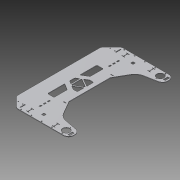
# Autodesk Inventor part: Shell
Saved by Autodesk Inventor 2015 (Build 190159000, 159)
## iProperties
Created: 2011-09-21
Part Number: Shell
Document SubType Name: Modeling
Designer: user
Density: 0.899 g/cm^3
Material: Polypropylene
Appearance: Smooth - White
Author: user
Autodesk Inventor part; units mm, degrees
ref_plane "YZ Plane" through (0, 0, 0) normal (1, 0, 0) x (0, 1, 0)
ref_plane "XZ Plane" through (0, 0, 0) normal (0, 1, 0) x (-1, 0, 0)
ref_plane "XY Plane" through (0, 0, 0) normal (0, 0, 1) x (1, 0, 0)
sketch "Profile" plane through (0, 0, 0) normal (0, 1, 0) x (-1, 0, 0)
  line L0 (-100, 0) -> (-164.5111, -37.2455)
  line L1 (-200.5386, -133.0137) -> (-188.6082, -71.0879)
  line L2 (-225.0872, -153.2843) -> (-230, -153.2843)
  arc A0 (-164.5111, -37.2455) -> (-188.6082, -71.0879) centre (-139.5111, -80.5468) ccw
  arc A1 (-225.0872, -153.2843) -> (-200.5386, -133.0137) centre (-225.0872, -128.2843) ccw
  arc A2 (-255, -128.2843) -> (-230, -153.2843) centre (-230, -128.2843) ccw
  line L3 (-100, 0) -> (0, 0)
  line L4 (-153, 47) -> (-143, 47)
  line L5 (-143, 47) -> (-143, 53)
  line L6 (-143, 53) -> (-153, 53)
  line L7 (-153, 53) -> (-153, 47)
  line L8 (-249.1421, 105.8579) -> (-210.8579, 144.1421)
  line L9 (-196.7157, 150) -> (0, 150)
  arc A3 (-249.1421, 105.8579) -> (-255, 91.7157) centre (-235, 91.7157) ccw
  arc A4 (-196.7157, 150) -> (-210.8579, 144.1421) centre (-196.7157, 130) ccw
  line L10 (0, 0) -> (0, 150) construction
  line L11 (-255, -128.2843) -> (-255, 91.7157)
  line L12 (-224.5, 102.5) -> (-221.5, 102.5)
  line L13 (-221.5, 102.5) -> (-221.5, 99.5)
  line L14 (-221.5, 99.5) -> (-224.5, 99.5)
  line L15 (-224.5, 99.5) -> (-224.5, 102.5)
  line L16 (-224.5, 124.5) -> (-221.5, 124.5)
  line L17 (-221.5, 124.5) -> (-221.5, 121.5)
  line L18 (-221.5, 121.5) -> (-224.5, 121.5)
  line L19 (-224.5, 121.5) -> (-224.5, 124.5)
  line L20 (-40, 25) -> (-40, 38.7438)
  arc A5 (-39.2646, 41.354) -> (-40, 38.7438) centre (-35, 38.7438) ccw
  arc A6 (-40, 25) -> (-35, 20) centre (-35, 25) ccw
  line L21 (-5.7735, 20) -> (-35, 20)
  line L22 (-114, 0) -> (-115, 0)
  line L23 (-116, 1) -> (-116, 11)
  line L24 (-115, 12) -> (-114, 12)
  line L25 (-113, 11) -> (-113, 1)
  line L26 (-211, 12) -> (-221, 12)
  line L27 (-222, 11) -> (-222, 1)
  line L28 (-221, 0) -> (-211, 0)
  line L29 (-210, 1) -> (-210, 11)
  arc A7 (-113, 11) -> (-114, 12) centre (-114, 11) ccw
  arc A8 (-114, 0) -> (-113, 1) centre (-114, 1) ccw
  arc A9 (-116, 1) -> (-115, 0) centre (-115, 1) ccw
  arc A10 (-115, 12) -> (-116, 11) centre (-115, 11) ccw
  arc A11 (-221, 12) -> (-222, 11) centre (-221, 11) ccw
  arc A12 (-210, 11) -> (-211, 12) centre (-211, 11) ccw
  arc A13 (-211, 0) -> (-210, 1) centre (-211, 1) ccw
  arc A14 (-222, 1) -> (-221, 0) centre (-221, 1) ccw
  line L30 (-247.5, -142.5) -> (-215.5, -142.5) construction
  line L31 (100, 0) -> (164.5111, -37.2455)
  line L32 (200.5386, -133.0137) -> (188.6082, -71.0879)
  line L33 (225.0872, -153.2843) -> (230, -153.2843)
  arc A15 (188.6082, -71.0879) -> (164.5111, -37.2455) centre (139.5111, -80.5468) ccw
  arc A16 (200.5386, -133.0137) -> (225.0872, -153.2843) centre (225.0872, -128.2843) ccw
  arc A17 (230, -153.2843) -> (255, -128.2843) centre (230, -128.2843) ccw
  line L34 (100, 0) -> (0, 0)
  line L35 (153, 47) -> (143, 47)
  line L36 (143, 47) -> (143, 53)
  line L37 (143, 53) -> (153, 53)
  line L38 (153, 53) -> (153, 47)
  line L39 (249.1421, 105.8579) -> (210.8579, 144.1421)
  arc A18 (255, 91.7157) -> (249.1421, 105.8579) centre (235, 91.7157) ccw
  arc A19 (210.8579, 144.1421) -> (196.7157, 150) centre (196.7157, 130) ccw
  line L40 (255, -128.2843) -> (255, 91.7157)
  line L41 (224.5, 102.5) -> (221.5, 102.5)
  line L42 (221.5, 102.5) -> (221.5, 99.5)
  line L43 (221.5, 99.5) -> (224.5, 99.5)
  line L44 (224.5, 99.5) -> (224.5, 102.5)
  line L45 (224.5, 124.5) -> (221.5, 124.5)
  line L46 (221.5, 124.5) -> (221.5, 121.5)
  line L47 (221.5, 121.5) -> (224.5, 121.5)
  line L48 (224.5, 121.5) -> (224.5, 124.5)
  line L49 (40, 25) -> (40, 38.7438)
  arc A20 (40, 38.7438) -> (39.2646, 41.354) centre (35, 38.7438) ccw
  arc A21 (35, 20) -> (40, 25) centre (35, 25) ccw
  line L50 (5.7735, 20) -> (35, 20)
  line L51 (114, 0) -> (115, 0)
  line L52 (116, 1) -> (116, 11)
  line L53 (115, 12) -> (114, 12)
  line L54 (113, 11) -> (113, 1)
  line L55 (211, 12) -> (221, 12)
  line L56 (222, 11) -> (222, 1)
  line L57 (221, 0) -> (211, 0)
  line L58 (210, 1) -> (210, 11)
  arc A22 (114, 12) -> (113, 11) centre (114, 11) ccw
  arc A23 (113, 1) -> (114, 0) centre (114, 1) ccw
  arc A24 (115, 0) -> (116, 1) centre (115, 1) ccw
  arc A25 (116, 11) -> (115, 12) centre (115, 11) ccw
  arc A26 (222, 11) -> (221, 12) centre (221, 11) ccw
  arc A27 (211, 12) -> (210, 11) centre (211, 11) ccw
  arc A28 (210, 1) -> (211, 0) centre (211, 1) ccw
  arc A29 (221, 0) -> (222, 1) centre (221, 1) ccw
  line L59 (-247.5, -142.5) -> (-247.5, 96.5) construction
  line L60 (-215.5, -142.5) -> (-215.5, 96.5) construction
  line L61 (-215.5, 96.5) -> (-247.5, 96.5) construction
  circle A30 centre (-250, -117.5) radius 2.5
  circle A31 centre (-250, -67.5) radius 2.5
  circle A32 centre (-250, -17.5) radius 2.5
  circle A33 centre (-250, 32.5) radius 2.5
  circle A34 centre (-250, 82.5) radius 2.5
  circle A35 centre (250, -117.5) radius 2.5
  circle A36 centre (250, -67.5) radius 2.5
  circle A37 centre (250, -17.5) radius 2.5
  circle A38 centre (250, 32.5) radius 2.5
  circle A39 centre (250, 82.5) radius 2.5
  line L62 (-173, 47) -> (-163, 47)
  line L63 (-163, 47) -> (-163, 53)
  line L64 (-163, 53) -> (-173, 53)
  line L65 (-173, 53) -> (-173, 47)
  line L66 (-193, 47) -> (-183, 47)
  line L67 (-183, 47) -> (-183, 53)
  line L68 (-183, 53) -> (-193, 53)
  line L69 (-193, 53) -> (-193, 47)
  line L70 (173, 47) -> (163, 47)
  line L71 (163, 53) -> (173, 53)
  line L72 (173, 53) -> (173, 47)
  line L73 (163, 47) -> (163, 53)
  line L74 (193, 47) -> (183, 47)
  line L75 (183, 53) -> (193, 53)
  line L76 (193, 53) -> (193, 47)
  line L77 (183, 47) -> (183, 53)
  line L78 (196.7157, 150) -> (0, 150)
  line L79 (-25.4034, 64) -> (25.4034, 64)
  line L80 (-25.4034, 64) -> (0, 20)
  line L81 (25.4034, 64) -> (0, 20)
  line L82 (-28.3745, 59.146) -> (-5.7735, 20)
  line L83 (28.3745, 59.146) -> (5.7735, 20)
  line L84 (-39.2646, 41.354) -> (-28.3745, 59.146)
  line L85 (39.2646, 41.354) -> (28.3745, 59.146)
  line L86 (-22.343, 69) -> (22.343, 69)
  line L87 (22.343, 69) -> (14.9249, 81.1195)
  line L88 (8, 85) -> (-8, 85)
  line L89 (-14.9249, 81.1195) -> (-22.343, 69)
  arc A40 (-8, 85) -> (-14.9249, 81.1195) centre (-8, 76.8809) ccw
  arc A41 (14.9249, 81.1195) -> (8, 85) centre (8, 76.8809) ccw
  point P0 (-184.2881, -48.6637)
  point P1 (-204.4439, -153.2843)
  point P2 (-205, 150)
  point P3 (-223, 121.5)
  point P4 (-223, 102.5)
  point P5 (0, 20)
  point P6 (-116, 12)
  point P7 (-116, 0)
  point P8 (-113, 12)
  point P9 (-210, 12)
  point P10 (-222, 12)
  point P11 (-210, 0)
  point P12 (184.2881, -48.6637)
  point P13 (204.4439, -153.2843)
  point P14 (205, 150)
  point P15 (223, 121.5)
  point P16 (223, 102.5)
  point P17 (40, 20)
  point P18 (40, 40)
  point P19 (116, 12)
  point P20 (116, 0)
  point P21 (113, 12)
  point P22 (210, 12)
  point P23 (222, 12)
  point P24 (210, 0)
  point P25 (-114.5, 0)
  point P26 (0, 85)
  dimension "d595" = 12
  dimension "d646" = 100
  dimension "d649" = 5
  dimension "d653" = 50
  dimension "d658" = 239
  dimension "d659" = 32
  dimension "d660" = 5
  dimension "d665" = 150
  dimension "d666" = 50
  dimension "d668" = 220
  dimension "d673" = 13
  dimension "d675" = 3
  dimension "d677" = 1
  dimension "d678" = 12
  dimension "d679" = 43
  dimension "d680" = 6
  dimension "d681" = 10
  dimension "d682" = 47
  dimension "d686" = 20
  dimension "d691" = 25
  dimension "d695" = 20
  dimension "d699" = 3
  dimension "d703" = 3
  dimension "d708" = 5
  dimension "d710" = 150
  dimension "d711" = 58.2843
  dimension "d713" = 5
  dimension "d714" = 33
  dimension "d716" = 45
  dimension "d717" = 130.905
  dimension "d720" = 54.4614
  dimension "d722" = 155
  dimension "d738" = 25
  dimension "d759" = 20
  dimension "d760" = 80
  dimension "d762" = 60
  dimension "d767" = 5
  dimension "d768" = 5
  dimension "d769" = 148.53
  dimension "d774" = 5
  dimension "d775" = 16
  dimension "d777" = 65
  dimension "d779" = 16
  dimension "d780" = 21.354
  dimension "d796" = 25
  dimension "d798" = 3
  dimension "d799" = 25.5
  dimension "d800" = 30.5
  constraints: 180 end point, 83 symmetric about line, 64 point on circle, 42 centre point, 39 point on line, 35 tangent, 13 parallel, 12 horizontal, 10 equal radius, 8 perpendicular, 6 collinear, 6 horizontal alignment, 4 midpoint, 4 vertical, 2 coincident, 45 other
  measures "d595" distance of point (-116, 0) point (-116, 12)
  measures "d646" distance of L0.start L3.end
  measures "d649" diameter of A30
  measures "d653" distance of A30.centre A31.centre
  measures "d658" distance of L30.end L60.end
  measures "d659" distance of L30.start L30.end
  measures "d660" radius of A6
  measures "d665" angle of L3 L0
  measures "d666" radius of A0
  measures "d668" distance of L11.start L11.end
  measures "d673" distance from line of L0.start L25
  measures "d675" distance between parallel lines of L25 L23
  measures "d677" radius of A7
  measures "d678" distance between parallel lines of L29 L27
  measures "d679" distance from line of L0.start L5
  measures "d680" distance of L4.end L5.end
  measures "d681" distance of L5.end L6.end
  measures "d682" distance between parallel lines of L3 L4
  measures "d686" distance of L4.end L62.end
  measures "d691" radius of A2
  measures "d695" radius of A4
  measures "d699" distance of L16.end L17.end
  measures "d703" distance between parallel lines of L61 L14
  measures "d708" radius of A5
  measures "d710" distance between parallel lines of L3 L9
  measures "d711" distance from line of L9 L11.end
  measures "d713" distance from line of L11 A30.centre
  measures "d714" distance between parallel lines of L11 L27
  measures "d716" angle of L8 L9
  measures "d717" angle of L1 L0
  measures "d720" horizontal distance of L11.start L1.start
  measures "d722" distance from line of L0.start L11
  measures "d738" distance from line of L30 A30.centre
  measures "d759" distance between parallel lines of L3 L21
  measures "d760" distance between parallel lines of L49 L20
  measures "d762" angle of L81 L79
  measures "d767" distance between parallel lines of L82 L80
  measures "d768" distance between parallel lines of L81 L83
  measures "d769" angle of L20 L84
  measures "d774" distance between parallel lines of L79 L86
  measures "d775" distance between parallel lines of L86 L88
  measures "d777" distance between parallel lines of L50 L88
  measures "d779" distance of L88.start L88.end
  measures "d780" distance from line of L21 L84.start
  measures "d796" distance between parallel lines of L14 L16
  measures "d798" distance of L16.start L16.end
  measures "d799" distance between parallel lines of L9 L16
  measures "d800" distance between parallel lines of L11 L19
extrude "Extrusion22" add sketch "Profile" along normal blind 3
sketch "Sketch40" plane through (0, 3, 0) normal (0, 1, 0) x (1, 0, 0)
  line L0 (255, -91.7157) -> (255, 128.2843) projected
  line L1 (-255, 128.2843) -> (-255, -91.7157) projected
  circle A0 centre (207.5, 114.5) radius 1.5
  circle A1 centre (250, 117.5) radius 2.5 projected
  circle A2 centre (-250, 117.5) radius 2.5 projected
  line L2 (0, 0) -> (0, 165.3372) construction
  circle A3 centre (228, 114.5) radius 17.5
  circle A4 centre (-207.5, 114.5) radius 1.5
  circle A5 centre (-228, 114.5) radius 17.5
  dimension "d742" = 5
  dimension "d749" = 5
  dimension "d624" = 3
  dimension "d754" = 35
  dimension "d755" = 20.5
  dimension "d757" = 27
  dimension "d758" = 3
  constraints: 4 centre point, 3 vertical, 2 end point, 2 symmetric about line, 1 horizontal alignment, 2 other
  measures "d624" diameter of A0
  measures "d754" diameter of A3
  measures "d755" distance of A0.centre A3.centre
  measures "d757" distance from line of L0 A3.centre
  measures "d758" vertical distance of A1.centre A3.centre
extrude "Extrusion23" cut sketch "Sketch40" against normal through all contours A0 | A3 | A4 | A5
sketch "Sketch41" plane through (0, 3, 0) normal (0, 1, 0) x (1, 0, 0)
  line L0 (35.9987, -85) -> (55.5853, -53)
  line L1 (55.5853, -53) -> (120, -53)
  line L2 (120, -53) -> (120, -85)
  line L3 (120, -85) -> (35.9987, -85)
  line L4 (39.2646, -41.354) -> (28.3745, -59.146) projected
  line L5 (100, 0) -> (-100, 0) projected
  line L6 (-196.7157, -150) -> (196.7157, -150) projected
  line L7 (0, 0) -> (0, -150) construction
  line L8 (-35.9987, -85) -> (-55.5853, -53)
  line L9 (-55.5853, -53) -> (-120, -53)
  line L10 (-120, -53) -> (-120, -85)
  line L11 (-120, -85) -> (-35.9987, -85)
  point P0 (18.7058, -74.7898)
  point P1 (28.3745, -59.146)
  dimension "d630" = 20
  dimension "d631" = 53
  dimension "d633" = 85
  dimension "d731" = 20
  constraints: 18 end point, 4 symmetric about line, 2 perpendicular, 1 horizontal, 1 midpoint, 2 other
  measures "d631" distance between parallel lines of L5 L1
  measures "d633" distance between parallel lines of L5 L3
  measures "d731" distance from line of L5.start L2
extrude "Extrusion24" cut sketch "Sketch41" against normal through all
fillet "Fillet15" radius 5 6 edges at (120, 1.5, 85) (120, 1.5, 53) (55.5853, 1.5, 53) (-120, 1.5, 53) (-120, 1.5, 85) (-55.5853, 1.5, 53)
fillet "Fillet16" radius 2 2 edges at (-35.9987, 1.5, 85) (35.9987, 1.5, 85)
sketch "Sketch44" plane through (0, 3, 0) normal (0, 1, 0) x (1, 0, 0)
  line L0 (247.5, -94.5) -> (215.5, -94.5) construction
  line L1 (215.5, -94.5) -> (215.5, 145.5) construction
  line L2 (215.5, 145.5) -> (247.5, 145.5) construction
  line L3 (247.5, 145.5) -> (247.5, -94.5) construction
  circle A0 centre (250, -82.5) radius 2.5 construction
  line L4 (224.5, -99.5) -> (221.5, -99.5) construction
  line L5 (243.5, -64) -> (243.5, -51)
  line L6 (243.5, -64) -> (241.5, -64)
  line L7 (241.5, -64) -> (241.5, -58.5)
  line L8 (241.5, -58.5) -> (221.5, -58.5)
  line L9 (221.5, -58.5) -> (221.5, -64)
  line L10 (221.5, -64) -> (219.5, -64)
  line L11 (219.5, -64) -> (219.5, -51)
  line L12 (219.5, -51) -> (221.5, -51)
  line L13 (221.5, -51) -> (221.5, -56.5)
  line L14 (221.5, -56.5) -> (241.5, -56.5)
  line L15 (241.5, -56.5) -> (241.5, -51)
  line L16 (243.5, -51) -> (241.5, -51)
  circle A1 centre (250, -32.5) radius 2.5 construction
  line L17 (250, -82.5) -> (250, -32.5) construction
  circle A2 centre (250, 17.5) radius 2.5 construction
  line L18 (250, -32.5) -> (250, 17.5) construction
  line L19 (243.5, 74) -> (243.5, 61)
  line L20 (243.5, 74) -> (241.5, 74)
  line L21 (241.5, 74) -> (241.5, 68.5)
  line L22 (241.5, 68.5) -> (221.5, 68.5)
  line L23 (221.5, 68.5) -> (221.5, 74)
  line L24 (221.5, 74) -> (219.5, 74)
  line L25 (219.5, 74) -> (219.5, 61)
  line L26 (219.5, 61) -> (221.5, 61)
  line L27 (221.5, 61) -> (221.5, 66.5)
  line L28 (221.5, 66.5) -> (241.5, 66.5)
  line L29 (241.5, 66.5) -> (241.5, 61)
  line L30 (243.5, 61) -> (241.5, 61)
  line L31 (-196.7157, -150) -> (196.7157, -150) construction
  line L32 (0, -150) -> (0, 0) construction
  line L33 (-243.5, -64) -> (-243.5, -51)
  line L34 (-243.5, -64) -> (-241.5, -64)
  line L35 (-241.5, -64) -> (-241.5, -58.5)
  line L36 (-241.5, -58.5) -> (-221.5, -58.5)
  line L37 (-221.5, -58.5) -> (-221.5, -64)
  line L38 (-221.5, -64) -> (-219.5, -64)
  line L39 (-219.5, -64) -> (-219.5, -51)
  line L40 (-219.5, -51) -> (-221.5, -51)
  line L41 (-221.5, -51) -> (-221.5, -56.5)
  line L42 (-221.5, -56.5) -> (-241.5, -56.5)
  line L43 (-241.5, -56.5) -> (-241.5, -51)
  line L44 (-243.5, -51) -> (-241.5, -51)
  line L45 (-241.5, 68.5) -> (-221.5, 68.5)
  line L46 (-221.5, 66.5) -> (-241.5, 66.5)
  line L47 (-219.5, 74) -> (-219.5, 61)
  line L48 (-221.5, 68.5) -> (-221.5, 74)
  line L49 (-221.5, 74) -> (-219.5, 74)
  line L50 (-219.5, 61) -> (-221.5, 61)
  line L51 (-221.5, 61) -> (-221.5, 66.5)
  line L52 (-241.5, 74) -> (-241.5, 68.5)
  line L53 (-241.5, 66.5) -> (-241.5, 61)
  line L54 (-243.5, 61) -> (-241.5, 61)
  line L55 (-243.5, 74) -> (-243.5, 61)
  line L56 (-243.5, 74) -> (-241.5, 74)
  line L57 (243.5, -95) -> (219.5, -95)
  line L58 (219.5, -95) -> (219.5, -91)
  line L59 (219.5, -91) -> (243.5, -91)
  line L60 (243.5, -91) -> (243.5, -95)
  line L61 (242.5, 136) -> (220.5, 136)
  line L62 (220.5, 136) -> (220.5, 146)
  line L63 (220.5, 146) -> (242.5, 146)
  line L64 (242.5, 146) -> (242.5, 136)
  line L65 (-247.5, 145.5) -> (-247.5, -94.5) construction
  line L66 (-224.5, -99.5) -> (-221.5, -99.5) construction
  line L67 (-243.5, -95) -> (-219.5, -95)
  line L68 (-219.5, -95) -> (-219.5, -91)
  line L69 (-219.5, -91) -> (-243.5, -91)
  line L70 (-243.5, -91) -> (-243.5, -95)
  line L71 (-242.5, 136) -> (-220.5, 136)
  line L72 (-220.5, 136) -> (-220.5, 146)
  line L73 (-220.5, 146) -> (-242.5, 146)
  line L74 (-242.5, 146) -> (-242.5, 136)
  circle A3 centre (250, 67.5) radius 2.5 projected
  point P0 (250, -57.5)
  point P1 (243.5, -57.5)
  point P2 (-250, -57.5)
  point P3 (-243.5, -57.5)
  point P4 (231.5, -95)
  point P5 (231.5, -94.5)
  point P6 (231.5, 146)
  point P7 (231.5, 145.5)
  point P8 (-215.5, 145.5)
  point P9 (-231.5, -95)
  point P10 (-231.5, -94.5)
  point P11 (-231.5, 146)
  point P12 (-231.5, 145.5)
  point P13 (243.5, 67.5)
  dimension "d723" = 32
  dimension "d724" = 240
  dimension "d725" = 5
  dimension "d726" = 2
  dimension "d727" = 2
  dimension "d728" = 13
  dimension "d732" = 24
  dimension "d733" = 4
  dimension "d734" = 0.5
  dimension "d735" = 22
  dimension "d736" = 10
  dimension "d737" = 0.5
  dimension "d794" = 4
  dimension "d795" = 4
  constraints: 146 end point, 43 symmetric about line, 20 point on line, 10 perpendicular, 8 equal length, 8 horizontal, 8 midpoint, 6 parallel, 5 collinear, 4 vertical, 2 horizontal alignment, 2 vertical alignment, 1 tangent
  measures "d723" distance of L1.end L2.end
  measures "d724" distance of L0.end L1.end
  measures "d725" distance between parallel lines of L4 L0
  measures "d726" distance of L11.end L12.end
  measures "d727" distance between parallel lines of L14 L8
  measures "d728" distance of L10.end L11.end
  measures "d732" distance of L58.end L59.end
  measures "d733" distance of L57.end L58.end
  measures "d734" distance between parallel lines of L0 L57
  measures "d735" distance of L62.end L63.end
  measures "d736" distance of L61.end L62.end
  measures "d737" distance between parallel lines of L2 L63
  measures "d794" distance between parallel lines of L3 L5
  measures "d795" distance between parallel lines of L1 L11
extrude "Extrusion25" cut sketch "Sketch44" against normal through all contours L6 L7 L8 L9 L10 L11 L12 L13 L14 L15 L16 L5 | L19 L30 L29 L28 L27 L26 L25 L24 L23 L22 L21 L20 | L33 L44 L43 L42 L41 L40 L39 L38 L37 L36 L35 L34 | L45 L48 L49 L47 L50 L51 L46 L53 L54 L55 L56 L52 | L57 L58 L59 L60 | L61 L62 L63 L64 | L70 L69 L68 L67 | L74 L73 L72 L71
fillet "Fillet18" radius 2 9 edges at (25.4034, 1.5, 64) (28.3745, 1.5, 59.146) (5.7735, 1.5, 20) (0, 1.5, 20) (-5.7735, 1.5, 20) (-25.4034, 1.5, 64) (-28.3745, 1.5, 59.146) (22.343, 1.5, 69) (-22.343, 1.5, 69)
sketch "Sketch42" plane through (0, 0, 0) normal (0, -1, 0) x (1, 0, 0)
  line L0 (100, 0) -> (100, 150)
  line L1 (-196.7157, 150) -> (196.7157, 150) projected
  point P0 (0, 0)
  constraints: 2 end point, 1 point on line, 1 vertical
sketch "Sketch43" plane through (-151.1747, -250.7604, 91.7157) normal (0.7071068, -0.7071068, 0) x (-0.7071068, -0.7071068, 0)
  line L0 (-155, 91.7157) -> (-155, -58.2843)
  line L1 (-58.2843, -58.2843) -> (-354.2146, -58.2843) projected
  point P0 (-284.211, 91.7157)
  constraints: 2 end point, 1 point on line, 1 vertical
body "Solid11"
